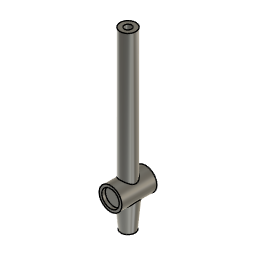
wind_speed_shaft (Autodesk Fusion 360 design; units mm, degrees)
Autodesk Fusion 360 part; units mm, degrees
sketch "Szkic1" plane through (0, 0, 0) normal (0, 0, 1) x (1, 0, 0)
sketch "Szkic2" plane through (0, 0, 0) normal (0, 0, 1) x (1, 0, 0)
  circle A0 centre (0, 0) radius 4.525
  dimension "d1" = 9.05
  constraint coincident A0.centre origin
  measures "d1" diameter of A0
extrude "Wyciągnięcie proste1" add sketch "Szkic2" along normal blind 100
sketch "Szkic3" plane through (0, 0, 0) normal (0, 1, 0) x (1, 0, 0)
  circle A0 centre (0, -20) radius 6.5
  circle A1 centre (0, -20) radius 5
  dimension "d4" = 13
  dimension "d5" = 10
  dimension "d6" = 20
  constraint concentric A0 A1
  measures "d4" diameter of A0
  measures "d5" diameter of A1
  measures "d6" distance of A0.centre origin
extrude "Wyciągnięcie proste2" add sketch "Szkic3" along normal mid plane 20
extrude "Wyciągnięcie proste3" add sketch "Szkic3" along normal mid plane 16 contours A1
sketch "Szkic4" plane through (0, 0, 100) normal (0, 0, 1) x (-1, 0, 0)
  circle A0 centre (0, 0) radius 4.525
  circle A1 centre (0, 0) radius 2.05
  dimension "d11" = 4.1
  constraint concentric A0 A1
  measures "d11" diameter of A1
extrude "Wyciągnięcie proste4" cut sketch "Szkic4" against normal blind 8 contours A1
draft "Draft1" angle 5 neutral plane through (0, 0, 0) pull (0, 0, -1) 1 faces at (4.5129, -0.3309, 5.1077)
move_face "OffsetFaces1" offset -0.5 1 faces at (4.3823, -3.6823, 13.7043)
ref_plane "WorkPlane1" through (0, -4.525, 30.8515) normal (0, -1, 0) x (-1, 0, 0)
